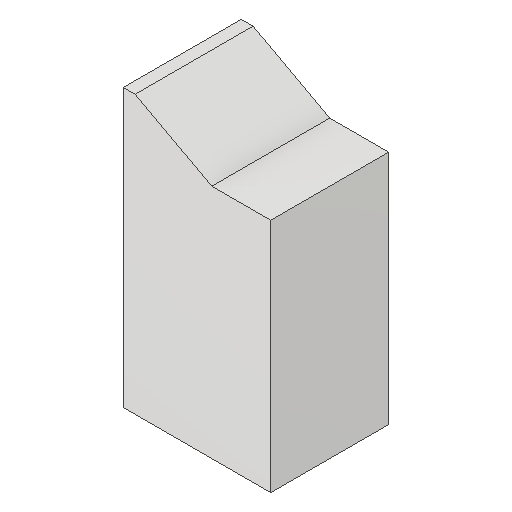
# Autodesk Inventor part: 3DP_PLA_Pick_up_tray
Saved by Autodesk Inventor 2026.1 (Build 301233000, 233)
## iProperties
Created: 2018-08-02
Part Number: 3DP_PLA_Pick_up_tray
Material: ABS Plastic
Document SubType Name: Modeling
Designer: Andrzej
Density: 1.06 g/cm^3
Appearance: Smooth - White
Author: Andrzej
Autodesk Inventor part; units mm, degrees
ref_plane "YZ Plane" through (0, 0, 0) normal (1, 0, 0) x (0, 1, 0)
ref_plane "XZ Plane" through (0, 0, 0) normal (0, 1, 0) x (-1, 0, 0)
ref_plane "XY Plane" through (0, 0, 0) normal (0, 0, 1) x (1, 0, 0)
sketch "Sketch1" plane through (0, 0, 0) normal (0, 0, 1) x (1, 0, 0)
  line L0 (-7.3355, -16.4371) -> (17.6645, -16.4371)
  line L1 (17.6645, -16.4371) -> (17.6645, 23.5629)
  line L2 (-7.3355, -16.4371) -> (-7.3355, 30.5629)
  line L3 (17.6645, 23.5629) -> (7.6645, 23.5629)
  line L4 (7.6645, 23.5629) -> (-5.3355, 30.5629)
  line L5 (-5.3355, 30.5629) -> (-7.3355, 30.5629)
  point P0 (0, 0)
  dimension "d0" = 25
  dimension "d1" = 2
  dimension "d2" = 10
  dimension "d5" = 40
  dimension "d6" = 47
  constraints: 12 end point, 2 horizontal, 1 parallel, 1 perpendicular, 1 vertical
  measures "d0" distance of L0.start L0.end
  measures "d1" distance of L4.end L2.end
  measures "d2" distance of L1.end L3.end
  measures "d5" distance of L0.end L1.end
  measures "d6" distance of L0.start L2.end
extrude "Extrusion1" add sketch "Sketch1" along normal blind 20
body "Solid1"
